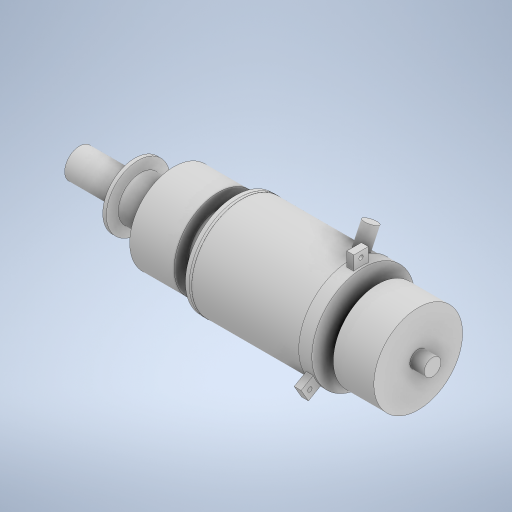
# Autodesk Inventor part: STI Hybrid 98 Cryocooler
Saved by Autodesk Inventor 2023 (Build 270158000, 158)
## iProperties
Created: 2024-04-30
Part Number: STI Hybrid 98 Cryocooler
Material: Generic
Document SubType Name: Modeling
Designer: incep
Density: 1 g/cm^3
Appearance: Default
Author: incep
Autodesk Inventor part; units mm, degrees
ref_plane "YZ Plane" through (0, 0, 0) normal (1, 0, 0) x (0, 1, 0)
sketch "Sketch1" plane through (0, 0, 0) normal (0, 1, 0) x (-1, 0, 0)
  line L0 (0, 0) -> (-303.89, 0)
  line L1 (0, 0) -> (0, -12.7)
  line L2 (0, -12.7) -> (-87.53, -12.7)
  line L3 (-87.53, -12.7) -> (-87.53, -17.315)
  line L4 (-87.53, -17.315) -> (-50.03, -17.315)
  line L5 (-50.03, -17.315) -> (-50.03, -20.525)
  line L6 (-50.03, -20.525) -> (-47.53, -20.525)
  line L7 (-47.53, -20.525) -> (-47.53, -27.45)
  line L8 (-47.53, -27.45) -> (-50.63, -27.45)
  line L9 (-50.63, -27.45) -> (-52.53, -19.05)
  line L10 (-52.53, -19.05) -> (-81.13, -19.05)
  line L11 (-81.13, -19.05) -> (-81.13, -37.85)
  line L12 (-81.13, -37.85) -> (-119.39, -37.85)
  line L13 (-119.39, -37.85) -> (-119.39, -25.55)
  line L14 (-119.39, -25.55) -> (-134.29, -37.635)
  line L15 (-134.29, -37.635) -> (-134.29, -43.07)
  line L16 (-134.29, -43.07) -> (-137.79, -43.07)
  line L17 (-137.79, -43.07) -> (-137.79, -43.28)
  line L18 (-137.79, -43.28) -> (-139.89, -43.28)
  line L19 (-139.89, -43.28) -> (-139.89, -43.175)
  line L20 (-139.89, -43.175) -> (-233.04, -43.175)
  line L21 (-233.04, -43.175) -> (-233.04, -44.315)
  line L22 (-233.04, -44.315) -> (-244.34, -44.315)
  line L23 (-244.34, -44.315) -> (-244.34, 0)
  line L24 (-256.65, 0) -> (-256.65, -38.15)
  line L25 (-256.65, -38.15) -> (-291.54, -38.15)
  line L26 (-291.54, -38.15) -> (-291.54, -7.165)
  line L27 (-291.54, -7.165) -> (-303.89, -7.165)
  line L28 (-303.89, -7.165) -> (-303.89, 0)
  dimension "d0" = 303.89
  dimension "d1" = 12.7
  dimension "d2" = 87.53
  dimension "d3" = 4.615
  dimension "d4" = 37.5
  dimension "d5" = 3.21
  dimension "d6" = 2.5
  dimension "d7" = 27.45
  dimension "d8" = 3.1
  dimension "d9" = 5
  dimension "d10" = 19.05
  dimension "d11" = 30.5
  dimension "d12" = 37.85
  dimension "d13" = 38.26
  dimension "d14" = 12.3
  dimension "d16" = 14.9
  dimension "d17" = 37.635
  dimension "d18" = 43.07
  dimension "d19" = 3.5
  dimension "d20" = 43.28
  dimension "d21" = 2.1
  dimension "d22" = 43.175
  dimension "d23" = 98.75
  dimension "d24" = 44.315
  dimension "d25" = 110.05
  dimension "d26" = 12.31
  dimension "d27" = 157.25
  dimension "d28" = 38.15
  dimension "d29" = 90
  dimension "d30" = 7.165
  dimension "d31" = 12.35
  constraints: 58 end point, 12 perpendicular, 9 vertical, 3 horizontal, 2 parallel, 2 point on line
  measures "d0" distance of L0.start L0.end
  measures "d1" distance of L0.start L1.end
  measures "d2" distance of L1.end L2.end
  measures "d3" distance of L2.end L3.end
  measures "d4" distance of L3.end L4.end
  measures "d5" distance of L4.end L5.end
  measures "d6" distance of L5.end L6.end
  measures "d7" vertical distance of L0.start L7.end
  measures "d8" distance of L7.end L8.end
  measures "d9" distance from line of L9.end L7
  measures "d10" distance from line of L10 L0.start
  measures "d11" distance from line of L11 L8.end
  measures "d12" distance from line of L0.start L12
  measures "d13" distance of L11.end L12.end
  measures "d14" distance of L12.end L13.end
  measures "d16" distance between parallel lines of L15 L13
  measures "d17" distance from line of L14.end L0
  measures "d18" distance between parallel lines of L0 L16
  measures "d19" distance of L15.end L16.end
  measures "d20" distance between parallel lines of L0 L18
  measures "d21" distance of L17.end L18.end
  measures "d22" distance between parallel lines of L0 L20
  measures "d23" distance from line of L20.end L15
  measures "d24" distance between parallel lines of L0 L22
  measures "d25" distance between parallel lines of L23 L15
  measures "d26" distance between parallel lines of L24 L23
  measures "d27" distance from line of L25.end L15
  measures "d28" distance between parallel lines of L0 L25
  measures "d29" angle of L27 L26
  measures "d30" distance of L27.end L0.end
  measures "d31" distance of L26.end L27.end
revolve "Revolution1" add sketch "Sketch1" angle 360 about axis through (0, 0, 0) along (1, 0, 0)
ref_plane "Work Plane1" through (242.34, 0, 0) normal (1, 0, 0) x (0, 0, -1)
sketch "Sketch3" plane through (242.34, 0, 0) normal (1, 0, 0) x (0, 0, -1)
  circle A0 centre (0, 0) radius 44.315 projected
  line L0 (-6.3, 55.8649) -> (6.3, 55.8649)
  line L1 (6.3, 55.8649) -> (6.3, 43.8649)
  line L2 (6.3, 43.8649) -> (-6.3, 43.8649)
  line L3 (-6.3, 43.8649) -> (-6.3, 55.8649)
  circle A1 centre (0, 50.8) radius 1.85
  line L4 (-6.3, 44.315) -> (6.3, 44.315) construction
  line L5 (124.271, 70.9929) -> (36.131, 70.9929)
  line L6 (36.131, 70.9929) -> (80.201, 147.3244)
  line L7 (80.201, 147.3244) -> (124.271, 70.9929)
  circle A2 centre (80.201, 96.4367) radius 50.8877
  circle A3 centre (0, 0) radius 50.8 construction
  point P0 (0, 55.8649)
  point P1 (0, 44.315)
  point P2 (19.1143, 39.9808)
  dimension "d51" = 101.7753
  dimension "d53" = 101.6
  dimension "d35" = 12.6
  dimension "d36" = 12
  dimension "d37" = 3.7
  dimension "d45" = 13.39
  dimension "d50" = 88.14
  constraints: 16 end point, 3 point on circle, 3 vertical alignment, 2 coincident, 2 horizontal, 2 midpoint, 2 parallel, 2 perpendicular, 2 point on line, 1 centre point, 1 tangent, 12 other
  measures "d35" distance of L0.start L0.end
  measures "d36" distance of L0.end L1.end
  measures "d37" diameter of A1
  measures "d45" distance of point (19.114, 39.981) L1.end
  measures "d50" distance of L5.start L5.end
extrude "Extrusion1" add sketch "Sketch3" against normal blind 6 contours A0 L3 L0 L1
pattern_circular "Circular Pattern1" count 3 over 360 about axis through (-10, 0, 0) along (1, 0, 0) of "Extrusion1"
ref_plane "Work Plane2" through (242.34, 39.9808, -19.1143) normal (0, 0.9021954, -0.4313276) x (-1, 0, 0)
sketch "Sketch5" plane through (242.34, 39.9808, -19.1143) normal (0, 0.9021954, -0.4313276) x (-1, 0, 0)
  circle A0 centre (18.085, 0) radius 6
  line L0 (-2, 44.315) -> (-2, -44.315) projected
  point P0 (242.34, 0)
  point P1 (0, 0)
  dimension "d46" = 12
  dimension "d47" = 20.085
  constraints: 1 centre point, 1 horizontal alignment
  measures "d46" diameter of A0
  measures "d47" distance from line of A0.centre L0
extrude "Extrusion2" add sketch "Sketch5" along normal mid plane 34
body "Solid1"
